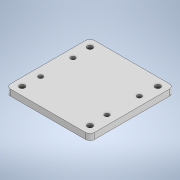
# Autodesk Inventor part: bottom
Saved by Autodesk Inventor 2020 (Build 240168000, 168)
## iProperties
Created: 2022-08-25
Part Number: bottom
Material: Типовые
Document SubType Name: Modeling
Designer: zigma
Density: 1 g/cm^3
Appearance: По умолчанию
Author: zigma
Autodesk Inventor part; units mm, degrees
ref_plane "YZ Plane" through (0, 0, 0) normal (1, 0, 0) x (0, 1, 0)
ref_plane "XZ Plane" through (0, 0, 0) normal (0, 1, 0) x (-1, 0, 0)
ref_plane "XY Plane" through (0, 0, 0) normal (0, 0, 1) x (1, 0, 0)
sketch "Эскиз1" plane through (0, 0, 0) normal (0, 1, 0) x (-1, 0, 0)
  line L0 (0, 0) -> (54.5, 0)
  line L1 (54.5, 0) -> (54.5, -54.5)
  line L2 (54.5, -54.5) -> (0, -54.5)
  line L3 (0, -54.5) -> (0, 0)
  dimension "d0" = 54.5
  dimension "d1" = 54.5
  constraints: 8 end point, 2 parallel, 1 horizontal, 1 perpendicular
  measures "d0" distance of L1.end L2.end
  measures "d1" distance of L0.end L1.end
extrude "Выдавливание1" add sketch "Эскиз1" along normal blind 4
fillet "Сопряжение1" radius 3 4 edges at (0, 2, 0) (0, 2, -54.5) (-54.5, 2, -54.5) (-54.5, 2, 0)
sketch "Эскиз2" plane through (0, 0, 0) normal (0, -1, 0) x (1, 0, 0)
  arc A0 (-54.5, -51.5) -> (-51.5, -54.5) centre (-51.5, -51.5) ccw projected
  line L0 (-54.5, -51.5) -> (-54.5, -3) projected
  line L1 (-54.5, -27.25) -> (0, -27.25) construction
  line L2 (0, -3) -> (0, -51.5) projected
  line L3 (-3, -54.5) -> (-51.5, -54.5) projected
  line L4 (-27.25, -54.5) -> (-27.25, 0) construction
  line L5 (-51.5, 0) -> (-3, 0) projected
  line L6 (-54.5, -51.5) -> (-54.5, -3) projected
  circle A1 centre (-49.25, -49.25) radius 3
  circle A2 centre (-49.25, -5.25) radius 3
  circle A3 centre (-5.25, -49.25) radius 3
  circle A4 centre (-5.25, -5.25) radius 3
  point P0 (0, 0)
  dimension "d13" = 6
  dimension "d34" = 44
  dimension "d35" = 44
  constraints: 4 centre point, 4 end point, 4 midpoint, 3 symmetric about line, 2 other
  measures "d13" diameter of A1
  measures "d34" distance of A2.centre A1.centre
  measures "d35" distance of A3.centre A1.centre
extrude "Выдавливание2" cut sketch "Эскиз2" against normal blind 2
sketch "Эскиз3" plane through (0, 2, 0) normal (0, -1, 0) x (1, 0, 0)
  circle A0 centre (-49.25, -49.25) radius 1.75
  line L0 (-54.5, -51.5) -> (-54.5, -3) projected
  line L1 (-54.5, -27.25) -> (0, -27.25) construction
  line L2 (0, -3) -> (0, -51.5) projected
  line L3 (-3, -54.5) -> (-51.5, -54.5) projected
  line L4 (-27.25, -54.5) -> (-27.25, 0) construction
  line L5 (-51.5, 0) -> (-3, 0) projected
  circle A1 centre (-49.25, -5.25) radius 1.75
  circle A2 centre (-5.25, -49.25) radius 1.75
  circle A3 centre (-5.25, -5.25) radius 1.75
  circle A4 centre (-49.25, -49.25) radius 3 construction
  circle A5 centre (-49.25, -49.25) radius 3
  point P0 (0, 0)
  point P1 (-45.0293, -48.6853)
  point P2 (-51.4707, -47.8147)
  dimension "d9" = 3.5
  constraints: 5 centre point, 4 end point, 4 midpoint, 3 symmetric about line, 2 coincident, 3 other
  measures "d9" diameter of A0
extrude "Выдавливание3" cut sketch "Эскиз3" against normal blind 2 contours A0 | A1 | A2 | A3
sketch "Эскиз4" plane through (0, 4, 0) normal (0, 1, 0) x (1, 0, 0)
  line L0 (-54.5, 51.5) -> (-54.5, 3) projected
  line L1 (-54.5, 12.5) -> (0, 12.5) construction
  line L2 (0, 3) -> (0, 51.5) construction
  line L3 (-54.5, 42) -> (0, 42) construction
  line L4 (-51.5, 0) -> (-3, 0) projected
  line L5 (-3, 54.5) -> (-51.5, 54.5) projected
  line L6 (-52, 14.5) -> (-2.5, 14.5) construction
  line L7 (-2.5, 14.5) -> (-2.5, 40) construction
  line L8 (-2.5, 40) -> (-52, 40) construction
  line L9 (-52, 40) -> (-52, 14.5) construction
  line L10 (-48.75, 16.75) -> (-5.75, 16.75) construction
  line L11 (-5.75, 16.75) -> (-5.75, 37.75) construction
  line L12 (-5.75, 37.75) -> (-48.75, 37.75) construction
  line L13 (-48.75, 37.75) -> (-48.75, 16.75) construction
  line L14 (-27.25, 14.5) -> (-27.25, 40) construction
  line L15 (-2.5, 27.25) -> (-27.25, 27.25) construction
  line L16 (-27.25, 16.75) -> (-27.25, 37.75) construction
  line L17 (-5.75, 27.25) -> (-27.25, 27.25) construction
  circle A0 centre (-48.75, 16.75) radius 1.5
  circle A1 centre (-48.75, 37.75) radius 1.5
  circle A2 centre (-5.75, 37.75) radius 1.5
  circle A3 centre (-5.75, 16.75) radius 1.5
  line L18 (-27.25, 12.5) -> (-27.25, 42) construction
  line L19 (-27.25, 27.25) -> (-21.7344, 27.25) construction
  point P0 (0, 0)
  dimension "d15" = 12.5
  dimension "d16" = 12.5
  dimension "d17" = 49.5
  dimension "d18" = 25.5
  dimension "d19" = 43
  dimension "d20" = 21
  dimension "d21" = 3
  dimension "d22" = 3
  dimension "d23" = 3
  dimension "d24" = 3
  constraints: 32 end point, 11 midpoint, 5 horizontal, 4 centre point, 4 parallel, 2 perpendicular, 2 point on line, 1 coincident
  measures "d15" distance between parallel lines of L4 L1
  measures "d16" distance between parallel lines of L5 L3
  measures "d17" distance of L8.end L7.end
  measures "d18" distance of L7.end L6.end
  measures "d19" distance of L12.end L11.end
  measures "d20" distance of L11.end L10.end
  measures "d21" diameter of A0
  measures "d22" diameter of A1
  measures "d23" diameter of A2
  measures "d24" diameter of A3
extrude "Выдавливание4" cut sketch "Эскиз4" against normal blind 4
sketch "Эскиз5" plane through (0, 0, 0) normal (0, -1, 0) x (1, 0, 0)
  circle A0 centre (-5.75, -16.75) radius 1.5 projected
  circle A1 centre (-5.75, -16.75) radius 2.25
  line L0 (-3.5, -16.75) -> (-4.625, -18.6986)
  line L1 (-4.625, -18.6986) -> (-6.875, -18.6986)
  line L2 (-6.875, -18.6986) -> (-8, -16.75)
  line L3 (-8, -16.75) -> (-6.875, -14.8014)
  line L4 (-6.875, -14.8014) -> (-4.625, -14.8014)
  line L5 (-4.625, -14.8014) -> (-3.5, -16.75)
  circle A2 centre (-5.75, -37.75) radius 1.5 projected
  circle A3 centre (-5.75, -37.75) radius 1.5
  circle A4 centre (-48.75, -37.75) radius 1.5 projected
  circle A5 centre (-48.75, -37.75) radius 1.5
  circle A6 centre (-48.75, -16.75) radius 1.5 projected
  circle A7 centre (-48.75, -16.75) radius 1.5
  line L6 (-3.5, -37.75) -> (-4.625, -39.6986)
  line L7 (-4.625, -39.6986) -> (-6.875, -39.6986)
  line L8 (-6.875, -39.6986) -> (-8, -37.75)
  line L9 (-8, -37.75) -> (-6.875, -35.8014)
  line L10 (-6.875, -35.8014) -> (-4.625, -35.8014)
  line L11 (-4.625, -35.8014) -> (-3.5, -37.75)
  line L12 (-46.5, -37.75) -> (-47.625, -39.6986)
  line L13 (-47.625, -39.6986) -> (-49.875, -39.6986)
  line L14 (-49.875, -39.6986) -> (-51, -37.75)
  line L15 (-51, -37.75) -> (-49.875, -35.8014)
  line L16 (-49.875, -35.8014) -> (-47.625, -35.8014)
  line L17 (-47.625, -35.8014) -> (-46.5, -37.75)
  line L18 (-46.5, -16.75) -> (-47.625, -18.6986)
  line L19 (-47.625, -18.6986) -> (-49.875, -18.6986)
  line L20 (-49.875, -18.6986) -> (-51, -16.75)
  line L21 (-51, -16.75) -> (-49.875, -14.8014)
  line L22 (-49.875, -14.8014) -> (-47.625, -14.8014)
  line L23 (-47.625, -14.8014) -> (-46.5, -16.75)
  point P0 (0, 0)
  dimension "d27" = 4.5
  constraints: 48 end point, 5 coincident, 3 centre point, 1 horizontal alignment, 15 other
extrude "Выдавливание5" cut sketch "Эскиз5" against normal blind 2 contours A0 | L0 L1 L2 L3 L4 L5 | A2 | A4 | A6 | L6 L7 L8 L9 L10 L11 | L12 L13 L14 L15 L16 L17 | L18 L19 L20 L21 L22 L23
equation "\"d0\" = d1"
equation "\"d22\" = d21"
equation "\"d23\" = d21"
equation "\"d24\" = d21"
